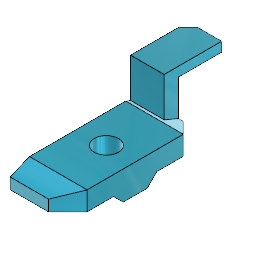
Endstop Flag X V2 (Autodesk Fusion 360 design; units mm, degrees)
Autodesk Fusion 360 part; units mm, degrees
ref_plane "WorkPlane2" through (38.5, 10, 36) normal (1, 0, 0) x (0, 1, 0)
sketch "Sketch3" plane through (38.5, 254.143, 26) normal (1, 0, 0) x (0, 1, 0)
  line L0 (14.8526, -10) -> (18.8526, -10)
  line L1 (18.8526, -10) -> (18.8526, 8.3252)
  line L2 (18.8526, 8.3252) -> (14.8526, 10)
  line L3 (14.8526, 10) -> (-5.1474, 10)
  line L4 (-5.1474, 10) -> (-9.1474, 8.3252)
  line L5 (-9.1474, 8.3252) -> (-9.1474, -10)
  line L6 (-9.1474, -10) -> (-5.1474, -10)
  line L7 (-5.1474, -10) -> (-5.1474, 6)
  line L8 (-5.1474, 6) -> (14.8526, 6)
  line L9 (14.8526, 6) -> (14.8526, -10)
  line L10 (-9.1474, 6) -> (18.8526, 6)
  line L11 (4.8526, 6) -> (4.8526, 4) construction
  line L12 (0.3526, 6) -> (2.3526, 4)
  line L13 (2.3526, 4) -> (7.3526, 4)
  line L14 (7.3526, 4) -> (9.3526, 6)
  dimension "d6958" = 2
  dimension "d6959" = 45
  dimension "d6960" = 5
  measures "d6959" angle of L10 L12
extrude "Extrude4" add sketch "Sketch3" along normal blind 12 contours L1 L2 L3 L4 L5 L8 L10 | L8 L10 L12 L13 L14
hole "Hole1" at (44.5, 258.9957, 36) direction (0, 0, -1) diameter 5 depth 14 tip angle 118
sketch "Sketch4" plane through (0, 272.9957, 0) normal (0, 1, 0) x (-1, 0, 0)
  line L0 (-38.5, 34.3252) -> (-38.5, 32)
  line L1 (-50.5, 34.3252) -> (-50.5, 32)
  line L2 (-38.5, 36) -> (-38.5, 34.3252)
  line L3 (-50.5, 36) -> (-50.5, 34.3252)
  line L4 (-38.5, 36) -> (-50.5, 36) construction
  line L5 (-50.5, 32) -> (-38.5, 32)
  line L6 (-38.5, 32) -> (-38.5, 43.75)
  line L7 (-38.5, 43.75) -> (-50.5, 43.75)
  line L8 (-50.5, 43.75) -> (-50.5, 32)
  line L9 (-38.5, 41.75) -> (-40.8835, 43.75)
  line L10 (-38.5, 41.75) -> (-50.5, 41.75)
  line L11 (-45.5, 43.75) -> (-45.5, 32)
  line L12 (-44.5, 30) -> (-50.5, 30)
  line L13 (-38.5, 30) -> (-44.5, 30)
  line L14 (-38.5, 32) -> (-38.5, 30)
  line L15 (-50.5, 32) -> (-50.5, 30)
  dimension "d6879" = 11.75
  dimension "d6880" = 2
  dimension "d6881" = 40
  dimension "d6889" = 7
  measures "d6881" angle of L9 L10
extrude "Extrude5" add sketch "Sketch4" against normal blind 3 contours L0 L2 L5 L6 L10 L11 | L6 L7 L9 | L7 L9 L10 L11
extrude "Extrude6" add sketch "Sketch4" along normal blind 9 contours L6 L7 L9 | L7 L9 L10 L11
chamfer "Chamfer7" distance 4 angle 45 2 edges at (50.5, 272.9957, 33.1626) (50.5, 244.9957, 33.1626)
chamfer "Chamfer8" distance 2 angle 45 1 edges at (38.5, 281.9957, 42.75)
named bodies: "X Endstop Flag V2"
